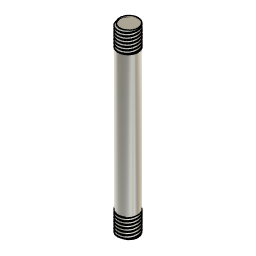
axle_twoside_threads v1 (Autodesk Fusion 360 design; units mm, degrees)
Autodesk Fusion 360 part; units mm, degrees
note: some values were not read from the file. Set by a fixed rule: which face or edge a step refers to.
sketch "Sketch1" plane through (0, 0, 0) normal (0, 0, 1) x (1, 0, 0)
  circle A0 centre (0, 0) radius 5
  dimension "d1" = 10
  constraint coincident A0.centre origin
  measures "d1" diameter of A0
extrude "Extrude1" add sketch "Sketch1" along normal blind 90 makes body 1
thread "Thread1" "ISO Metric profile 10.0 M10x1.5 M10x1.5 6g" major diameter 9.85 minor diameter 8.141 pitch 1.5 angle 60 modelled right hand crest width 0.2177 on face at (4.9938, -0.2492, 60) from (0, 0, 80) to (0, 0, 90) crest through (4.925, 0, -0.375) on bodies 1
copy_body "CopyPasteBodies1" bodies 1 makes body 2
move_body "Move1" bodies 2 to x (1, 0, 0) y (0, 1, 0) z (0, 0, 1) at (0, 35, 0)
sketch "Sketch2" plane through (0, 0, 0) normal (0, 0, -1) x (1, 0, 0)
  circle A0 centre (0, 0) radius 4.925
  line L0 (1.5, -3) -> (-1.5, -3)
  line L1 (-1.5, -3) -> (-1.5, 3)
  line L2 (-1.5, 3) -> (1.5, 3)
  line L3 (1.5, 3) -> (1.5, -3)
  line L4 (1.5, -3) -> (-1.5, 3) construction
  line L5 (-1.5, -3) -> (1.5, 3) construction
  dimension "d6" = 3
  dimension "d7" = 6
  constraint horizontal L0
  constraint perpendicular L0 L1
  constraint parallel L0 L2
  constraint parallel L1 L3
  constraint coincident L4 A0.centre
  constraint coincident L5 A0.centre
  constraint coincident A0.centre origin
  measures "d6" distance of L1.end L2.end
  measures "d7" distance of L0.end L1.end
extrude "Extrude2" cut sketch "Sketch2" against normal blind 10 contours L0 L1 L2 L3 bodies 1
sketch "Sketch3" plane through (0, 0, 0) normal (0, 0, 1) x (1, 0, 0)
  circle A0 centre (17.4353, 16.4847) radius 10
  circle A1 centre (17.4353, 16.4847) radius 5.5
  dimension "d10" = 20
  dimension "d11" = 11
  constraint concentric A0 A1
  measures "d10" diameter of A0
  measures "d11" diameter of A1
extrude "Extrude3" add sketch "Sketch3" along normal blind 10 separate body makes body 3
thread "Thread2" "ISO Metric profile 10.0 M10x1.5 M10x1.5 6H" major diameter 10.198 minor diameter 8.526 pitch 1.5 angle 60 modelled right hand crest width 0.4094 on face at (22.9285, 16.2106, 6.6667) crest through (21.6983, 16.4847, 0.375) on bodies 3
sketch "Sketch4" plane through (0, 0, 0) normal (0, 0, 1) x (1, 0, 0)
move_body "Move2" bodies 3 to x (1, 0, 0) y (0, 1, 0) z (0, 0, 1) at (-15, 0, 0)
thread "Thread3" "ISO Metric profile 10.0 M10x1.5 M10x1.5 6g" major diameter 9.85 minor diameter 8.141 pitch 1.5 angle 60 modelled right hand crest width 0.2177 on face at (-3.3337, 31.3748, 26.7278) from (0, 35, 0) to (0, 35, 10) crest through (4.925, 35, -0.375) on bodies 2
hidden bodies 1 3
